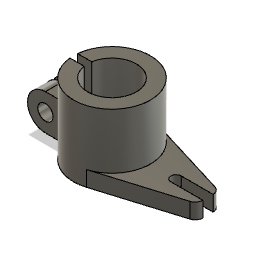
sample 1 (Autodesk Fusion 360 design; units mm, degrees)
Autodesk Fusion 360 part; units mm, degrees
sketch "Sketch1" plane through (0, 0, 0) normal (0, 1, 0) x (1, 0, 0)
  circle A0 centre (0, 0) radius 19
  circle A1 centre (0, 0) radius 30
  line L0 (0, 0) -> (50, 0) construction
  line L1 (50, 0) -> (75, 0) construction
  line L2 (50, 4) -> (75, 4)
  line L3 (50, -4) -> (75, -4)
  line L4 (8.7717, 28.689) -> (70.7543, 9.7378)
  arc A2 (75, 4) -> (70.7543, 9.7378) centre (69, 4) ccw
  arc A3 (50, 4) -> (50, -4) centre (50, 0) ccw
  line L5 (8.7717, -28.689) -> (70.7543, -9.7378)
  arc A4 (70.7543, -9.7378) -> (75, -4) centre (69, -4) ccw
  dimension "d1" = 38
  dimension "d2" = 60
  dimension "d3" = 50
  dimension "d4" = 8
  dimension "d5" = 25
  dimension "d6" = 4
  dimension "d7" = 4
  dimension "d8" = 12
  constraint coincident A0.centre A1.centre
  constraint horizontal L0
  constraint coincident L0.end L1.start
  constraint parallel L0 L1
  constraint tangent A1 L4
  constraint coincident L2 A2.centre
  constraint tangent L4 A2
  constraint coincident A1 L4.start
  constraint symmetric L0 L2.end L3.end
  constraint symmetric L0 L4.end L5.end
  constraint symmetric L0 A2 A4
  constraint symmetric L0 L4.start L5.start
  measures "d1" diameter of A0
  measures "d2" diameter of A1
  measures "d3" distance of A0.centre L0.end
  measures "d4" diameter of A3
  measures "d5" distance of L0.end L1.end
  measures "d8" diameter of A2
extrude "Extrude1" add sketch "Sketch1" along normal blind 44 contours A1
extrude "Extrude2" add sketch "Sketch1" along normal blind 12 contours A1 L2 L3 L4 A2 A3 L5 A4
sketch "Sketch2" plane through (0, 0, 0) normal (0, 0, 1) x (1, 0, 0)
  circle A0 centre (-36, 22) radius 6
  line L0 (-36, 36) -> (-22, 36)
  line L1 (-22, 36) -> (-22, 8)
  line L2 (-22, 8) -> (-36, 8)
  arc A1 (-36, 36) -> (-36, 8) centre (-36, 22) ccw
  line L3 (30, 0) -> (-30, 0)
  dimension "d14" = 28
  dimension "d15" = 12
  dimension "d16" = 8
  dimension "d17" = 36
  constraint concentric A0 A1
  constraint horizontal L0
  constraint vertical L1
  constraint horizontal L2
  constraint tangent L2 A1
  constraint tangent L1 A1
  measures "d14" diameter of A1
  measures "d15" diameter of A0
  measures "d16" distance of L2 L3
  measures "d17" horizontal distance of origin A0.centre
extrude "Extrude3" add sketch "Sketch2" along normal mid plane 32
sketch "Sketch3" plane through (0, 44, 0) normal (0, 1, 0) x (-1, 0, 0)
  circle A0 centre (0, 0) radius 19
  circle A1 centre (0, 0) radius 30
  line L0 (54, -3) -> (11, -3)
  line L1 (11, -3) -> (11, 3)
  line L2 (11, 3) -> (54, 3)
  line L3 (54, 3) -> (54, -3)
  line L4 (0, 0) -> (-50, 0)
  dimension "d20" = 3
  dimension "d21" = 3
  dimension "d22" = 11
  dimension "d23" = 43
  constraint horizontal L0
  constraint vertical L1
  constraint horizontal L2
  constraint vertical L3
  measures "d20" distance of L0 L4
  measures "d21" distance of L2 L4
  measures "d22" distance of A0.centre L1
  measures "d23" distance of L1 L3
extrude "Extrude4" cut sketch "Sketch3" against normal up to surface (44 mm away) contours A0 A1 L0 L2 | A1 L0 L2 L3
extrude "Extrude5" add 1 faces at (26.2783, 44, 0) along direction (0, 1, 0) blind 11.305
ref_plane "WorkPlane1" through (41.8858, 85.34, 0) normal (0, 1, 0) x (1, 0, 0)
ref_plane "WorkPlane2" through (0, 0, 57.35) normal (0, 0, 1) x (1, 0, 0)
